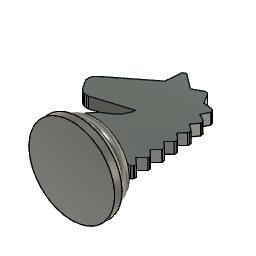
chess knight actual (Autodesk Fusion 360 design; units mm, degrees)
Autodesk Fusion 360 part; units mm, degrees
sketch "Sketch1" plane through (0, 0, 0) normal (0, 0, 1) x (1, 0, 0)
  line L0 (-1.0438, 10.1623) -> (2.8438, 7.2377)
  line L1 (2.8438, 7.2377) -> (5.4822, 8.7)
  line L2 (5.4822, 8.7) -> (5.8562, 8.7)
  line L3 (5.8562, 8.7) -> (6.1562, 8.5623)
  line L4 (6.1562, 8.5623) -> (6.3562, 8.3623)
  line L5 (6.3562, 8.3623) -> (8.0382, 5.6949)
  line L6 (8.0382, 5.6949) -> (10.541, 5.4625)
  line L7 (10.541, 5.4625) -> (10.8862, 5.2036)
  line L8 (10.8862, 5.2036) -> (11.0659, 4.8793)
  line L9 (11.0659, 4.8793) -> (11.0659, 4.5623)
  line L10 (11.0659, 4.5623) -> (10.1293, 2.5216)
  line L11 (10.1293, 2.5216) -> (11.9749, 1.4992)
  line L12 (11.9749, 1.4992) -> (12.2206, 1.227)
  line L13 (12.2206, 1.227) -> (12.3002, 0.8885)
  line L14 (12.3002, 0.8885) -> (12.2604, 0.603)
  line L15 (12.2604, 0.603) -> (10.9592, -1.1563)
  line L16 (10.9592, -1.1563) -> (12.8024, -2.5196)
  line L17 (12.8024, -2.5196) -> (12.8024, -3.0377)
  line L18 (12.8024, -3.0377) -> (12.7491, -3.4196)
  line L19 (12.7491, -3.4196) -> (11.3562, -4.8377)
  line L20 (11.3562, -4.8377) -> (11.3393, -4.9585)
  line L21 (11.3393, -4.9585) -> (12.9854, -6.3391)
  line L22 (12.9854, -6.3391) -> (13.0657, -6.5947)
  line L23 (13.0657, -6.5947) -> (13.0255, -6.9453)
  line L24 (13.0255, -6.9453) -> (12.9854, -7.2958)
  line L25 (12.9854, -7.2958) -> (11.5562, -8.6377)
  line L26 (11.5562, -8.6377) -> (13.1679, -10.1445)
  line L27 (13.1679, -10.1445) -> (13.2021, -10.6371)
  line L28 (13.2021, -10.6371) -> (13.1679, -10.8008)
  line L29 (13.1679, -10.8008) -> (11.6422, -12.4328)
  line L30 (11.6422, -12.4328) -> (13.1679, -13.9315)
  line L31 (13.1679, -13.9315) -> (13.2784, -14.301)
  line L32 (13.2784, -14.301) -> (13.2231, -14.6459)
  line L33 (13.2231, -14.6459) -> (11.5562, -16.2377)
  line L34 (11.5562, -16.2377) -> (13.2231, -17.7658)
  line L35 (13.2231, -17.7658) -> (13.2508, -18.2149)
  line L36 (13.2508, -18.2149) -> (13.1929, -18.576)
  line L37 (13.1929, -18.576) -> (12.7562, -18.8377)
  line L38 (12.7562, -18.8377) -> (-7.0438, -18.8377)
  line L39 (-7.0438, -18.8377) -> (-7.6673, -18.2662)
  line L40 (-7.6673, -18.2662) -> (-7.6673, -17.7497)
  line L41 (-7.6673, -17.7497) -> (-7.1652, -17.3969)
  line L42 (-7.1652, -17.3969) -> (-6.8438, -17.3969)
  line L43 (-6.8438, -17.3969) -> (-6.7402, -15.7848)
  line L44 (-6.7402, -15.7848) -> (-6.3231, -14.0925)
  line L45 (-6.3231, -14.0925) -> (-5.5692, -12.5045)
  line L46 (-5.5692, -12.5045) -> (-4.7832, -11.4859)
  line L47 (-4.7832, -11.4859) -> (-3.4438, -10.2377)
  line L48 (-3.4438, -10.2377) -> (-1.535, -8.9034)
  line L49 (-1.535, -8.9034) -> (-0.5068, -7.9451)
  line L50 (-0.5068, -7.9451) -> (-0.0799, -7.046)
  line L51 (-0.0799, -7.046) -> (0.3562, -6.0377)
  line L52 (0.3562, -6.0377) -> (0.4299, -5.1981)
  line L53 (0.4299, -5.1981) -> (-9.2438, -8.2377)
  line L54 (-9.2438, -8.2377) -> (-9.8438, -8.2377)
  line L55 (-9.8438, -8.2377) -> (-10.4427, -8.1851)
  line L56 (-10.4427, -8.1851) -> (-10.9056, -7.9849)
  line L57 (-10.9056, -7.9849) -> (-11.6438, -7.4377)
  line L58 (-11.6438, -7.4377) -> (-13.3922, -4.9365)
  line L59 (-13.3922, -4.9365) -> (-13.4438, -4.0377)
  line L60 (-13.4438, -4.0377) -> (-13.3922, -3.4502)
  line L61 (-13.3922, -3.4502) -> (-13.1243, -2.8802)
  line L62 (-13.1243, -2.8802) -> (-12.8837, -2.5754)
  line L63 (-12.8837, -2.5754) -> (-2.4438, 5.5623)
  line L64 (-2.4438, 5.5623) -> (-2.0701, 9.8149)
  line L65 (-2.0701, 9.8149) -> (-1.6122, 10.1719)
  line L66 (-1.6122, 10.1719) -> (-1.3425, 10.281)
  line L67 (-1.3425, 10.281) -> (-1.0438, 10.1623)
  constraint horizontal L2
  constraint perpendicular L1 L8
  constraint perpendicular L2 L9
  constraint perpendicular L3 L10
  constraint perpendicular L15 L16
  constraint vertical L17
  constraint parallel L14 L18
  constraint parallel L18 L20
  constraint parallel L23 L24
  constraint perpendicular L26 L29
  constraint perpendicular L19 L30
  constraint parallel L32 L36
  constraint horizontal L38
  constraint parallel L34 L39
  constraint perpendicular L38 L40
  constraint parallel L38 L42
  constraint parallel L47 L49
  constraint parallel L45 L50
  constraint horizontal L54
  constraint perpendicular L52 L55
  constraint perpendicular L51 L56
  constraint perpendicular L48 L58
  constraint parallel L52 L60
  constraint parallel L60 L64
  constraint parallel L63 L65
extrude "Extrude1" add sketch "Sketch1" along normal blind 3 makes body 1
sketch "Sketch2" plane through (0, 0, 3) normal (0, 0, 1) x (-1, 0, 0)
  line L0 (1.3425, -10.281) -> (1.6122, -10.1719)
  line L1 (1.6122, -10.1719) -> (2.0701, -9.8149)
  line L2 (2.0701, -9.8149) -> (2.4438, -5.5623)
  line L3 (2.4438, -5.5623) -> (12.8837, 2.5754)
  line L4 (12.8837, 2.5754) -> (13.1243, 2.8802)
  line L5 (13.1243, 2.8802) -> (13.3922, 3.4502)
  line L6 (13.3922, 3.4502) -> (13.4438, 4.0377)
  line L7 (13.4438, 4.0377) -> (13.3922, 4.9365)
  line L8 (13.3922, 4.9365) -> (11.6438, 7.4377)
  line L9 (11.6438, 7.4377) -> (10.9056, 7.9849)
  line L10 (10.9056, 7.9849) -> (10.4427, 8.1851)
  line L11 (10.4427, 8.1851) -> (9.8438, 8.2377)
  line L12 (9.8438, 8.2377) -> (9.2438, 8.2377)
  line L13 (9.2438, 8.2377) -> (-0.4299, 5.1981)
  line L14 (-0.4299, 5.1981) -> (-0.3562, 6.0377)
  line L15 (-0.3562, 6.0377) -> (0.0799, 7.046)
  line L16 (0.0799, 7.046) -> (0.5068, 7.9451)
  line L17 (0.5068, 7.9451) -> (1.535, 8.9034)
  line L18 (1.535, 8.9034) -> (3.4438, 10.2377)
  line L19 (3.4438, 10.2377) -> (4.7832, 11.4859)
  line L20 (4.7832, 11.4859) -> (5.5692, 12.5045)
  line L21 (5.5692, 12.5045) -> (6.3231, 14.0925)
  line L22 (6.3231, 14.0925) -> (6.7402, 15.7848)
  line L23 (6.7402, 15.7848) -> (6.8438, 17.3969)
  line L24 (6.8438, 17.3969) -> (7.1652, 17.3969)
  line L25 (7.1652, 17.3969) -> (7.6673, 17.7497)
  line L26 (7.6673, 17.7497) -> (7.6673, 18.2662)
  line L27 (7.6673, 18.2662) -> (7.0438, 18.8377)
  line L28 (7.0438, 18.8377) -> (-12.7562, 18.8377)
  line L29 (-12.7562, 18.8377) -> (-13.1929, 18.576)
  line L30 (-13.1929, 18.576) -> (-13.2508, 18.2149)
  line L31 (-13.2508, 18.2149) -> (-13.2231, 17.7658)
  line L32 (-13.2231, 17.7658) -> (-11.5562, 16.2377)
  line L33 (-11.5562, 16.2377) -> (-13.2231, 14.6459)
  line L34 (-13.2231, 14.6459) -> (-13.2784, 14.301)
  line L35 (-13.2784, 14.301) -> (-13.1679, 13.9315)
  line L36 (-13.1679, 13.9315) -> (-11.6422, 12.4328)
  line L37 (-11.6422, 12.4328) -> (-13.1679, 10.8008)
  line L38 (-13.1679, 10.8008) -> (-13.2021, 10.6371)
  line L39 (-13.2021, 10.6371) -> (-13.1679, 10.1445)
  line L40 (-13.1679, 10.1445) -> (-11.5562, 8.6377)
  line L41 (-11.5562, 8.6377) -> (-12.9854, 7.2958)
  line L42 (-12.9854, 7.2958) -> (-13.0657, 6.5947)
  line L43 (-13.0657, 6.5947) -> (-12.9854, 6.3391)
  line L44 (-12.9854, 6.3391) -> (-11.3393, 4.9585)
  line L45 (-11.3393, 4.9585) -> (-11.3562, 4.8377)
  line L46 (-11.3562, 4.8377) -> (-12.7491, 3.4196)
  line L47 (-12.7491, 3.4196) -> (-12.8024, 3.0377)
  line L48 (-12.8024, 3.0377) -> (-12.8024, 2.5196)
  line L49 (-12.8024, 2.5196) -> (-10.9592, 1.1563)
  line L50 (-10.9592, 1.1563) -> (-12.2604, -0.603)
  line L51 (-12.2604, -0.603) -> (-12.3002, -0.8885)
  line L52 (-12.3002, -0.8885) -> (-12.2206, -1.227)
  line L53 (-12.2206, -1.227) -> (-11.9749, -1.4992)
  line L54 (-11.9749, -1.4992) -> (-10.1293, -2.5216)
  line L55 (-10.1293, -2.5216) -> (-11.0659, -4.5623)
  line L56 (-11.0659, -4.5623) -> (-11.0659, -4.8793)
  line L57 (-11.0659, -4.8793) -> (-10.8862, -5.2036)
  line L58 (-10.8862, -5.2036) -> (-10.541, -5.4625)
  line L59 (-10.541, -5.4625) -> (-8.0382, -5.6949)
  line L60 (-8.0382, -5.6949) -> (-6.3562, -8.3623)
  line L61 (-6.3562, -8.3623) -> (-6.1562, -8.5623)
  line L62 (-6.1562, -8.5623) -> (-5.8562, -8.7)
  line L63 (-5.8562, -8.7) -> (-5.4822, -8.7)
  line L64 (-5.4822, -8.7) -> (-2.8438, -7.2377)
  line L65 (-2.8438, -7.2377) -> (1.0438, -10.1623)
  line L66 (1.0438, -10.1623) -> (1.3425, -10.281)
sketch "Sketch3" plane through (0, 0, 0) normal (0, 0, 1) x (1, 0, 0)
  line L0 (2.9991, -18.8378) -> (2.9991, -25)
  line L1 (2.9991, -25) -> (14.5791, -25)
  line L2 (14.5791, -25) -> (14.5791, -23)
  line L3 (14.5791, -23) -> (13.5791, -23)
  line L4 (2.9991, -18.8378) -> (12.3391, -18.8378)
  arc A0 (12.5518, -20.9911) -> (12.3391, -18.8378) centre (11.5791, -20) ccw
  arc A1 (13.5791, -23) -> (12.5518, -20.9911) centre (12.0791, -22.5) ccw
  constraint vertical L0
  constraint perpendicular L0 L1
  constraint perpendicular L1 L2
  constraint perpendicular L2 L3
  constraint perpendicular L0 L4
revolve "Revolve1" add sketch "Sketch3" angle 360 about axis through (2.9991, -18.8378, 0) along (0, -1, 0) separate body makes body 2
